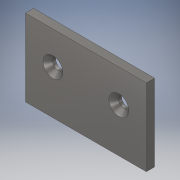
# Autodesk Inventor part: VS-003 (JAW PLATE)
Saved by Autodesk Inventor 2017 (Build 210142000, 142)
## iProperties
Created: 2016-11-30
Part Number: VS-003 (JAW PLATE)
Material: Steel, Alloy
Document SubType Name: Modeling
Designer: SCC
Density: 7.73 g/cm^3
Appearance: Semi-Polished
Author: SCC
Autodesk Inventor part; units mm, degrees
ref_plane "YZ Plane" through (0, 0, 0) normal (1, 0, 0) x (0, 1, 0)
ref_plane "XZ Plane" through (0, 0, 0) normal (0, 1, 0) x (-1, 0, 0)
ref_plane "XY Plane" through (0, 0, 0) normal (0, 0, 1) x (1, 0, 0)
sketch "Sketch1" plane through (0, 0, 0) normal (0, 0, 1) x (1, 0, 0)
  line L0 (0, 0) -> (69.85, 0)
  line L1 (69.85, 0) -> (69.85, 44.45)
  line L2 (69.85, 44.45) -> (0, 44.45)
  line L3 (0, 44.45) -> (0, 0)
  dimension "d0" = 69.85
  dimension "d1" = 44.45
  constraints: 8 end point, 2 parallel, 1 horizontal, 1 perpendicular
  measures "d0" distance of L0.start L0.end
  measures "d1" distance of L0.end L1.end
extrude "Extrusion1" add sketch "Sketch1" against normal blind 4.7625
hole "Hole1" at (15.875, 25.4, 0) direction (0, 0, -1) diameter 6.35 end through all countersink diameter 11.4808 countersink angle 82
hole "Hole2" at (53.975, 25.4, 0) direction (0, 0, -1) diameter 6.35 end through all countersink diameter 11.4808 countersink angle 82
body "Solid1"
